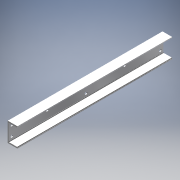
# Autodesk Inventor part: NASA-20-SP-01
Saved by Autodesk Inventor 2019 (Build 230136000, 136)
## iProperties
Created: 2019-09-05
Part Number: NASA-20-SP-01
Material: Aluminum 6061
Description: SIDE PLATE
Document SubType Name: Modeling
Designer: Rick Szalay
Stock Number: 1630T31
Density: 2.7 g/cm^3
Appearance: Aluminum - Flat
Author: Rick Szalay
Autodesk Inventor part; units mm, degrees
ref_plane "YZ Plane" through (0, 0, 0) normal (1, 0, 0) x (0, 1, 0)
ref_plane "XZ Plane" through (0, 0, 0) normal (0, 1, 0) x (-1, 0, 0)
ref_plane "XY Plane" through (0, 0, 0) normal (0, 0, 1) x (1, 0, 0)
sketch "Sketch3" plane through (0, 0, 0) normal (0, 0, 1) x (1, 0, 0)
  line L0 (0, 38.1) -> (0, -38.1)
  line L1 (0, 38.1) -> (38.1, 38.1)
  line L2 (38.1, 38.1) -> (38.1, 33.02)
  line L3 (38.1, 33.02) -> (3.302, 33.02)
  line L4 (3.302, 33.02) -> (3.302, -33.02)
  line L5 (3.302, -33.02) -> (38.1, -33.02)
  line L6 (38.1, -33.02) -> (38.1, -38.1)
  line L7 (38.1, -38.1) -> (0, -38.1)
  line L8 (0, 0) -> (3.302, 0) construction
  dimension "d7" = 76.2
  dimension "d8" = 3.302
  dimension "d9" = 66.04
  dimension "d10" = 38.1
  constraints: 18 end point, 6 perpendicular, 2 horizontal, 2 midpoint, 1 coincident, 1 vertical, 1 other
  measures "d7" distance of L0.start L0.end
  measures "d8" distance between parallel lines of L0 L4
  measures "d9" distance between parallel lines of L5 L3
  measures "d10" distance of L0.start L1.end
extrude "Extrusion3" add sketch "Sketch3" along normal mid plane 609.6
fillet "Fillet1" radius 3.175 4 edges at (38.1, 33.02, 0) (38.1, -33.02, 0) (3.302, -33.02, 0) (3.302, 33.02, 0)
sketch "Sketch4" plane through (0, -38.1, 304.8) normal (-1, 0, 0) x (0, 0, 1)
  line L0 (0, 76.2) -> (-609.6, 76.2) projected
  line L1 (-609.6, 0) -> (0, 0) projected
  line L2 (-609.6, 0) -> (-609.6, 76.2) projected
  line L3 (0, 76.2) -> (0, 0) projected
  point P0 (-304.8, 38.1)
  point P1 (-596.9, 19.05)
  point P2 (-596.9, 57.15)
  point P3 (-12.7, 19.05)
  point P4 (-12.7, 57.15)
  point P5 (-304.8, 19.05)
  point P6 (-304.8, 57.15)
  dimension "d14" = 19.05
  dimension "d15" = 19.05
  dimension "d16" = 12.7
  dimension "d24" = 12.7
  constraints: 4 horizontal alignment, 4 vertical alignment
  measures "d14" distance from line of point (-596.9, 57.15) L0
  measures "d15" distance from line of L1 point (-596.9, 19.05)
  measures "d16" distance from line of point (-596.9, 19.05) L2
  measures "d24" distance from line of point (-12.7, 57.15) L3
hole "Hole1" at (0, -19.05, -292.1) at (0, 19.05, -292.1) at (0, -19.05, 292.1) at (0, 19.05, 292.1) at (0, -19.05, 0) at (0, 19.05, 0) direction (1, 0, 0) diameter 10.0838 depth 25.4 tip angle 118 clearance for "Flat Head Machine Screw (82)" size "3/8" standard "Ansi Unified Screw Threads"
sketch "Sketch5" plane through (0, -38.1, 304.8) normal (-1, 0, 0) x (0, 0, 1)
  line L0 (-609.6, 0) -> (-609.6, 76.2) projected
  line L1 (-152.4, 38.1) -> (-304.8, 38.1) construction
  line L2 (-304.8, 38.1) -> (-457.2, 38.1) construction
  point P0 (-609.6, 38.1)
  dimension "d25" = 304.8
  constraints: 4 end point, 2 collinear, 2 horizontal alignment, 1 horizontal, 1 midpoint
  measures "d25" distance of L2.end L1.start
hole "Hole2" at (0, 0, -152.4) at (0, 0, 152.4) direction (1, 0, 0) diameter 10.0838 depth 25.4 tip angle 118 clearance for "Flat Head Machine Screw (82)" size "3/8" standard "Ansi Unified Screw Threads"
equation "\"d11\" = Length"
equation "\"Length\" = 609.6"
body "Solid2"
